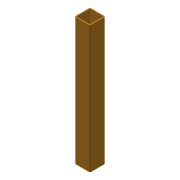
# Autodesk Inventor part: 3136 1094 43
Saved by Autodesk Inventor 2022 Beta2 (Build 260130000, 130) ContinuousBuild 0
## iProperties
Shininess: 64.0
Length Units: 11269
Angle Units: 11279
Time Units: 11290
Mass Units: 11283
Length Display Precision: 3
Angle Display Precision: 2
Compacted: True
Part Number: 3136 1094 43
Document SubType Name: Modeling
Created: 2003-04-13
Designer: Uffe Bak
Material: Steel, Mild
Density: 7.86 g/cm^3
Appearance: Brokk-Gul
Density: 0.0
Volumn: 0.0
Area: 0.0
PropertySet Name: Model Information
Control State: 0
Master: False
Checked Out: False
Author: Uffe Bak
Autodesk Inventor part; units mm, degrees
ref_plane "YZ Plane" through (0, 0, 0) normal (1, 0, 0) x (0, 1, 0)
ref_plane "XZ Plane" through (0, 0, 0) normal (0, 1, 0) x (-1, 0, 0)
ref_plane "XY Plane" through (0, 0, 0) normal (0, 0, 1) x (1, 0, 0)
sketch "Sketch1" plane through (0, 0, 0) normal (0, 0, 1) x (1, 0, 0)
  line L0 (40, 34) -> (40, -34)
  line L1 (34, -40) -> (-34, -40)
  line L2 (-40, -34) -> (-40, 34)
  line L3 (-34, 40) -> (34, 40)
  arc A0 (-34, 40) -> (-40, 34) centre (-34, 34) ccw
  arc A1 (40, 34) -> (34, 40) centre (34, 34) ccw
  arc A2 (34, -40) -> (40, -34) centre (34, -34) ccw
  arc A3 (-40, -34) -> (-34, -40) centre (-34, -34) ccw
  arc A4 (-34, 35) -> (-35, 34) centre (-34, 34) ccw
  line L4 (-34, 35) -> (34, 35)
  arc A5 (35, 34) -> (34, 35) centre (34, 34) ccw
  line L5 (35, 34) -> (35, -34)
  arc A6 (34, -35) -> (35, -34) centre (34, -34) ccw
  line L6 (34, -35) -> (-34, -35)
  arc A7 (-35, -34) -> (-34, -35) centre (-34, -34) ccw
  line L7 (-35, -34) -> (-35, 34)
  point P0 (0, 0)
  point P1 (0, 0)
  point P2 (40, 40)
  point P3 (40, -40)
  point P4 (-40, -40)
  point P5 (-40, 40)
  dimension "d0" = 80
  dimension "d1" = 6
  dimension "d2" = 6
  dimension "d3" = 6
  dimension "d4" = 6
  dimension "d5" = 5
  constraints: 16 end point, 16 point on circle, 8 centre point, 8 point on line, 8 tangent, 1 coincident, 14 other
  measures "d0" distance of point (-40, 40) point (40, 40)
  measures "d1" radius of A0
  measures "d2" radius of A1
  measures "d3" radius of A2
  measures "d4" radius of A3
  measures "d5" distance between parallel lines of L2 L7
extrude "Extrusion1" add sketch "Sketch1" along normal blind 655
sketch "Sketch2" plane through (-40, -34, 0) normal (-1, 0, 0) x (0, 0, 1)
  line L0 (0, 0) -> (0, 68) projected
  line L1 (0, 0) -> (655, 0) projected
  line L2 (0, 34) -> (229, 34)
  line L3 (229, 34) -> (229, 52.5)
  line L4 (229, 34) -> (229, 15.5)
  dimension "d8" = 229
  dimension "d9" = 18.5
  constraints: 6 end point, 2 coincident, 2 collinear, 1 midpoint, 1 parallel, 1 perpendicular
  measures "d8" distance of L2.start L2.end
  measures "d9" distance of L2.end L3.end
hole "Hole1" at (-40, 18.5, 229) at (-40, -18.5, 229) direction (1, 0, 0) diameter 10 depth 8 tip angle 118
body "Solid1"
